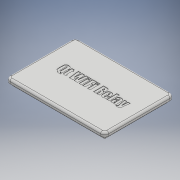
# Autodesk Inventor part: housing-lid
Saved by Autodesk Inventor 2018 (Build 220112000, 112)
## iProperties
Created: 2018-03-19
Part Number: housing-lid
Material: Generic
Document SubType Name: Modeling
Designer: matth
Density: 1 g/cm^3
Appearance: Default
Author: matth
Autodesk Inventor part; units mm, degrees
note: some values were not read from the file. Chosen so that the rebuilt part matches the saved one: direction of "Emboss1".
ref_plane "YZ Plane" through (0, 0, 0) normal (1, 0, 0) x (0, 1, 0)
ref_plane "XZ Plane" through (0, 0, 0) normal (0, 1, 0) x (-1, 0, 0)
ref_plane "XY Plane" through (0, 0, 0) normal (0, 0, 1) x (1, 0, 0)
sketch "Sketch1" plane through (0, 0, 0) normal (0, 0, 1) x (1, 0, 0)
  line L0 (0, 0) -> (46, 0)
  line L1 (46, 0) -> (46, 31.5)
  line L2 (46, 31.5) -> (0, 31.5)
  line L3 (0, 31.5) -> (0, 0)
  dimension "d0" = 46
  dimension "d1" = 31.5
  constraints: 8 end point, 2 parallel, 1 horizontal, 1 perpendicular
  measures "d0" distance of L1.end L2.end
  measures "d1" distance of L0.end L1.end
extrude "Extrusion1" add sketch "Sketch1" along normal blind 2
sketch "Sketch2" plane through (0, 0, 2) normal (0, 0, 1) x (1, 0, 0)
  line L0 (46, 0) -> (46, 31.5) projected
  line L1 (0, 0) -> (46, 0)
  line L2 (46, 0) -> (46, 31.5)
  line L3 (46, 31.5) -> (0, 31.5)
  line L4 (0, 31.5) -> (0, 0)
  line L5 (-1.4, 32.9) -> (47.4, 32.9)
  line L6 (47.4, 32.9) -> (47.4, -1.4)
  line L7 (47.4, -1.4) -> (-1.4, -1.4)
  line L8 (-1.4, -1.4) -> (-1.4, 32.9)
  dimension "d4" = 1.4
  constraints: 16 end point, 4 parallel, 2 perpendicular, 1 horizontal, 3 other
  measures "d4" distance between parallel lines of L3 L5
extrude "Extrusion2" add sketch "Sketch2" along normal blind 2 contours L1 L4 L3 L0 | L5 L6 L7 L8
sketch "Sketch3" plane through (0, 0, 0) normal (0, 0, -1) x (-1, 0, 0)
  line L0 (-46, 0) -> (-46, 31.5) projected
  line L1 (0, 0) -> (-46, 0)
  line L2 (-46, 0) -> (-46, 31.5)
  line L3 (-46, 31.5) -> (0, 31.5)
  line L4 (0, 31.5) -> (0, 0)
  line L5 (-43, 3) -> (-3, 3)
  line L6 (-3, 3) -> (-3, 28.5)
  line L7 (-3, 28.5) -> (-43, 28.5)
  line L8 (-43, 28.5) -> (-43, 3)
  dimension "d7" = 3
  constraints: 16 end point, 4 parallel, 2 perpendicular, 1 horizontal, 3 other
  measures "d7" distance between parallel lines of L1 L5
extrude "Extrusion3" cut sketch "Sketch3" against normal blind 2 contours L8 L7 L6 L5
chamfer "Chamfer1" distance 0.5 angle 45 4 edges at (23, 0, 0) (46, 15.75, 0) (23, 31.5, 0) (0, 15.75, 0)
chamfer "Chamfer2" distance 0.5 angle 45 4 edges at (0, 0, 1.25) (0, 31.5, 1.25) (46, 31.5, 1.25) (46, 0, 1.25)
fillet "Fillet1" radius 2 4 edges at (47.4, -1.4, 3) (47.4, 32.9, 3) (-1.4, 32.9, 3) (-1.4, -1.4, 3)
fillet "Fillet2" radius 1 8 edges at (46.8142, 32.3142, 4) (23, 32.9, 4) (-0.8142, 32.3142, 4) (-1.4, 15.75, 4) (-0.8142, -0.8142, 4) (23, -1.4, 4) (46.8142, -0.8142, 4) (47.4, 15.75, 4)
sketch "Sketch4" plane through (0, 0, 4) normal (0, 0, 1) x (1, 0, 0)
  line L0 (4.7033, 18.9978) -> (43.575, 18.9978) construction
  line L1 (43.575, 18.9978) -> (43.575, 6.6861) construction
  line L2 (43.575, 6.6861) -> (4.7033, 6.6861) construction
  line L3 (4.7033, 6.6861) -> (4.7033, 18.9978) construction
  line L4 (10.7801, 13.8923) -> (10.7801, 13.2857)
  line L5 (10.7801, 13.2857) -> (9.7967, 13.2857)
  spline S0 degree 2 poles (9.7967, 13.2857) (9.4425, 13.2857) (9.1524, 13.3949) (9.0506, 13.6135) (9.0506, 13.8923) knots 0 0 0 1 2 3 3 3
  spline S1 degree 2 poles (9.0506, 13.8923) (8.6098, 13.9036) (7.973, 14.3444) (7.7696, 15.0189) (7.7696, 15.6933) knots 0 0 0 1 2 3 3 3
  line L6 (7.7696, 15.6933) -> (7.7696, 17.242)
  spline S2 degree 2 poles (7.7696, 17.242) (7.7696, 17.7506) (7.8901, 18.2857) (8.2669, 18.7566) (8.8585, 18.9978) (9.2202, 18.9978) knots 0 0 0 1 2 3 4 4 4
  spline S3 degree 2 poles (9.2202, 18.9978) (9.6573, 18.9978) (10.3393, 18.7001) (10.6746, 18.2442) (10.7763, 17.7544) (10.7763, 17.2683) knots 0 0 0 1 2 3 4 4 4
  line L7 (10.7763, 17.2683) -> (10.7763, 15.6444)
  spline S4 degree 2 poles (10.7763, 15.6444) (10.7763, 14.9774) (10.6482, 14.5027) (10.279, 14.2201) (9.9738, 14.1485) knots 0 0 0 1 2 3 3 3
  spline S5 degree 2 poles (9.9738, 14.1485) (9.9813, 13.979) (10.1019, 13.8923) (10.328, 13.8923) knots 0 0 0 1 2 2 2
  line L8 (10.328, 13.8923) -> (10.7801, 13.8923)
  spline S6 degree 2 poles (9.4764, 17.6074) (9.4764, 17.9541) (9.4011, 18.15) (9.2805, 18.15) knots 0 0 0 1 2 2 2
  spline S7 degree 2 poles (9.2805, 18.15) (9.1787, 18.15) (9.0695, 17.9918) (9.0695, 17.6074) knots 0 0 0 1 2 2 2
  line L9 (9.0695, 17.6074) -> (9.0695, 15.2751)
  spline S8 degree 2 poles (9.0695, 15.2751) (9.0695, 14.838) (9.1411, 14.6346) (9.2692, 14.6346) knots 0 0 0 1 2 2 2
  spline S9 degree 2 poles (9.2692, 14.6346) (9.4011, 14.6346) (9.4764, 14.8682) (9.4764, 15.309) knots 0 0 0 1 2 2 2
  line L10 (9.4764, 15.309) -> (9.4764, 17.6074)
  line L11 (12.5397, 18.5381) -> (12.5397, 17.8938)
  line L12 (12.5397, 17.8938) -> (12.8788, 17.8938)
  line L13 (12.8788, 17.8938) -> (12.8788, 17.2457)
  line L14 (12.8788, 17.2457) -> (12.5397, 17.2457)
  line L15 (12.5397, 17.2457) -> (12.5397, 15.049)
  spline S10 degree 2 poles (12.5397, 15.049) (12.5397, 14.6459) (12.6226, 14.5517) (12.9316, 14.5517) knots 0 0 0 1 2 2 2
  line L16 (12.9316, 14.5517) -> (12.9316, 13.8923)
  line L17 (12.9316, 13.8923) -> (12.4267, 13.8923)
  spline S11 degree 2 poles (12.4267, 13.8923) (12.0009, 13.8923) (11.6354, 13.9639) (11.3566, 14.2201) (11.2888, 14.5517) (11.2888, 15.1621) knots 0 0 0 1 2 3 4 4 4
  line L18 (11.2888, 15.1621) -> (11.2888, 17.2457)
  line L19 (11.2888, 17.2457) -> (11.0212, 17.2457)
  line L20 (11.0212, 17.2457) -> (11.0212, 17.8938)
  line L21 (11.0212, 17.8938) -> (11.2888, 17.8938)
  line L22 (11.2888, 17.8938) -> (11.2888, 18.5381)
  line L23 (11.2888, 18.5381) -> (12.5397, 18.5381)
  line L24 (19.1976, 18.8923) -> (18.6173, 13.8923)
  line L25 (18.6173, 13.8923) -> (16.9971, 13.8923)
  spline S12 degree 2 poles (16.9971, 13.8923) (16.7748, 15.0453) (16.6053, 16.5147) knots 0 0 0 1 1 1
  spline S13 degree 2 poles (16.6053, 16.5147) (16.5224, 15.8855) (16.2398, 13.8923) knots 0 0 0 1 1 1
  line L26 (16.2398, 13.8923) -> (14.6271, 13.8923)
  line L27 (14.6271, 13.8923) -> (14.0469, 18.8923)
  line L28 (14.0469, 18.8923) -> (15.3091, 18.8923)
  line L29 (15.3091, 18.8923) -> (15.4448, 17.1478)
  line L30 (15.4448, 17.1478) -> (15.5804, 15.4597)
  spline S14 degree 2 poles (15.5804, 15.4597) (15.652, 16.771) (15.9384, 18.8923) knots 0 0 0 1 1 1
  line L31 (15.9384, 18.8923) -> (17.2873, 18.8923)
  spline S15 degree 2 poles (17.2873, 18.8923) (17.3136, 18.6738) (17.4267, 17.242) knots 0 0 0 1 1 1
  line L32 (17.4267, 17.242) -> (17.5736, 15.3392)
  spline S16 degree 2 poles (17.5736, 15.3392) (17.6867, 17.1553) (17.9353, 18.8923) knots 0 0 0 1 1 1
  line L33 (17.9353, 18.8923) -> (19.1976, 18.8923)
  line L34 (20.7047, 17.9918) -> (20.7047, 13.8923)
  line L35 (20.7047, 13.8923) -> (19.4199, 13.8923)
  line L36 (19.4199, 13.8923) -> (19.4199, 17.9918)
  line L37 (19.4199, 17.9918) -> (20.7047, 17.9918)
  line L38 (20.7047, 18.8923) -> (20.7047, 18.2404)
  line L39 (20.7047, 18.2404) -> (19.4199, 18.2404)
  line L40 (19.4199, 18.2404) -> (19.4199, 18.8923)
  line L41 (19.4199, 18.8923) -> (20.7047, 18.8923)
  line L42 (21.1908, 18.8923) -> (23.3913, 18.8923)
  line L43 (23.3913, 18.8923) -> (23.3913, 17.89)
  line L44 (23.3913, 17.89) -> (22.4907, 17.89)
  line L45 (22.4907, 17.89) -> (22.4907, 16.9443)
  line L46 (22.4907, 16.9443) -> (23.2933, 16.9443)
  line L47 (23.2933, 16.9443) -> (23.2933, 15.991)
  line L48 (23.2933, 15.991) -> (22.4907, 15.991)
  line L49 (22.4907, 15.991) -> (22.4907, 13.8923)
  line L50 (22.4907, 13.8923) -> (21.1908, 13.8923)
  line L51 (21.1908, 13.8923) -> (21.1908, 18.8923)
  line L52 (24.9549, 17.9918) -> (24.9549, 13.8923)
  line L53 (24.9549, 13.8923) -> (23.6701, 13.8923)
  line L54 (23.6701, 13.8923) -> (23.6701, 17.9918)
  line L55 (23.6701, 17.9918) -> (24.9549, 17.9918)
  line L56 (24.9549, 18.8923) -> (24.9549, 18.2404)
  line L57 (24.9549, 18.2404) -> (23.6701, 18.2404)
  line L58 (23.6701, 18.2404) -> (23.6701, 18.8923)
  line L59 (23.6701, 18.8923) -> (24.9549, 18.8923)
  line L60 (26.5563, 18.8923) -> (27.4757, 18.8923)
  spline S17 degree 2 poles (27.4757, 18.8923) (28.395, 18.8923) (29.0469, 18.7491) (29.4576, 18.1651) (29.4576, 17.5283) knots 0 0 0 1 2 3 3 3
  spline S18 degree 2 poles (29.4576, 17.5283) (29.4576, 16.9443) (29.1674, 16.5411) (28.7417, 16.4997) knots 0 0 0 1 2 2 2
  spline S19 degree 2 poles (28.7417, 16.4997) (29.126, 16.4055) (29.3935, 16.0852) (29.4576, 15.8177) (29.4576, 15.2111) knots 0 0 0 1 2 3 3 3
  line L61 (29.4576, 15.2111) -> (29.4576, 13.8923)
  line L62 (29.4576, 13.8923) -> (28.2481, 13.8923)
  line L63 (28.2481, 13.8923) -> (28.2481, 15.5539)
  spline S20 degree 2 poles (28.2481, 15.5539) (28.2481, 15.9533) (28.1237, 16.1455) (27.8562, 16.1455) knots 0 0 0 1 2 2 2
  line L64 (27.8562, 16.1455) -> (27.8562, 13.8923)
  line L65 (27.8562, 13.8923) -> (26.5563, 13.8923)
  line L66 (26.5563, 13.8923) -> (26.5563, 18.8923)
  line L67 (27.8562, 18.037) -> (27.8562, 16.9254)
  spline S21 degree 2 poles (27.8562, 16.9254) (28.0748, 16.9254) (28.2481, 17.046) (28.2481, 17.3776) knots 0 0 0 1 2 2 2
  line L68 (28.2481, 17.3776) -> (28.2481, 17.6527)
  spline S22 degree 2 poles (28.2481, 17.6527) (28.2481, 17.89) (28.0785, 18.037) (27.8562, 18.037) knots 0 0 0 1 2 2 2
  line L69 (32.7507, 15.8704) -> (31.1343, 15.8704)
  line L70 (31.1343, 15.8704) -> (31.1343, 14.985)
  spline S23 degree 2 poles (31.1343, 14.985) (31.1343, 14.7062) (31.2134, 14.5441) (31.3302, 14.5441) knots 0 0 0 1 2 2 2
  spline S24 degree 2 poles (31.3302, 14.5441) (31.4734, 14.5441) (31.5676, 14.7589) (31.5676, 15.0641) knots 0 0 0 1 2 2 2
  line L71 (31.5676, 15.0641) -> (31.5676, 15.6029)
  line L72 (31.5676, 15.6029) -> (32.7507, 15.6029)
  line L73 (32.7507, 15.6029) -> (32.7507, 15.3015)
  spline S25 degree 2 poles (32.7507, 15.3015) (32.7507, 14.9209) (32.6565, 14.514) (32.3023, 14.0505) (31.7635, 13.8169) (31.3528, 13.8169) knots 0 0 0 1 2 3 4 4 4
  spline S26 degree 2 poles (31.3528, 13.8169) (30.9572, 13.8169) (30.3543, 14.0468) (30.0152, 14.4462) (29.8871, 14.9247) (29.8871, 15.3806) knots 0 0 0 1 2 3 4 4 4
  line L74 (29.8871, 15.3806) -> (29.8871, 16.5788)
  spline S27 degree 2 poles (29.8871, 16.5788) (29.8871, 17.1138) (30.1772, 17.7355) (30.8404, 18.0671) (31.2662, 18.0671) knots 0 0 0 1 2 3 3 3
  spline S28 degree 2 poles (31.2662, 18.0671) (31.7937, 18.0671) (32.4757, 17.6677) (32.7507, 17.0121) (32.7507, 16.413) knots 0 0 0 1 2 3 3 3
  line L75 (32.7507, 16.413) -> (32.7507, 15.8704)
  line L76 (31.4998, 16.5374) -> (31.4998, 16.835)
  spline S29 degree 2 poles (31.4998, 16.835) (31.4998, 17.1553) (31.4319, 17.3399) (31.3264, 17.3399) knots 0 0 0 1 2 2 2
  spline S30 degree 2 poles (31.3264, 17.3399) (31.1946, 17.3399) (31.1343, 17.1817) (31.1343, 16.835) knots 0 0 0 1 2 2 2
  line L77 (31.1343, 16.835) -> (31.1343, 16.5374)
  line L78 (31.1343, 16.5374) -> (31.4998, 16.5374)
  line L79 (34.4425, 18.8923) -> (34.4425, 13.8923)
  line L80 (34.4425, 13.8923) -> (33.1576, 13.8923)
  line L81 (33.1576, 13.8923) -> (33.1576, 18.8923)
  line L82 (33.1576, 18.8923) -> (34.4425, 18.8923)
  line L83 (36.0062, 16.4055) -> (34.8344, 16.4055)
  line L84 (34.8344, 16.4055) -> (34.8344, 16.6805)
  spline S31 degree 2 poles (34.8344, 16.6805) (34.8344, 17.1553) (35.0529, 17.6715) (35.716, 18.0671) (36.2436, 18.0671) knots 0 0 0 1 2 3 3 3
  spline S32 degree 2 poles (36.2436, 18.0671) (36.8766, 18.0671) (37.5209, 17.6187) (37.649, 16.9669) (37.649, 15.9496) knots 0 0 0 1 2 3 3 3
  line L85 (37.649, 15.9496) -> (37.649, 13.8923)
  line L86 (37.649, 13.8923) -> (36.4357, 13.8923)
  line L87 (36.4357, 13.8923) -> (36.4357, 14.2578)
  spline S33 degree 2 poles (36.4357, 14.2578) (36.3227, 14.0392) (35.961, 13.8169) (35.7085, 13.8169) knots 0 0 0 1 2 2 2
  spline S34 degree 2 poles (35.7085, 13.8169) (35.3807, 13.8169) (34.8344, 14.1862) (34.8344, 14.8079) knots 0 0 0 1 2 2 2
  line L88 (34.8344, 14.8079) -> (34.8344, 15.1432)
  spline S35 degree 2 poles (34.8344, 15.1432) (34.8344, 15.6029) (35.1245, 15.9383) (35.701, 16.1606) knots 0 0 0 1 2 2 2
  spline S36 degree 2 poles (35.701, 16.1606) (36.3151, 16.4017) (36.4018, 16.5675) (36.4018, 16.8237) knots 0 0 0 1 2 2 2
  spline S37 degree 2 poles (36.4018, 16.8237) (36.4018, 17.144) (36.3076, 17.3399) (36.1946, 17.3399) knots 0 0 0 1 2 2 2
  spline S38 degree 2 poles (36.1946, 17.3399) (36.0665, 17.3399) (36.0062, 17.1779) (36.0062, 16.835) knots 0 0 0 1 2 2 2
  line L89 (36.0062, 16.835) -> (36.0062, 16.4055)
  spline S39 degree 2 poles (36.4018, 15.8441) (36.1004, 15.6255) (36.0062, 15.3279) (36.0062, 15.049) knots 0 0 0 1 2 2 2
  spline S40 degree 2 poles (36.0062, 15.049) (36.0062, 14.7288) (36.0891, 14.5441) (36.2134, 14.5441) knots 0 0 0 1 2 2 2
  spline S41 degree 2 poles (36.2134, 14.5441) (36.3302, 14.5441) (36.4018, 14.6911) (36.4018, 15.0001) knots 0 0 0 1 2 2 2
  line L90 (36.4018, 15.0001) -> (36.4018, 15.8441)
  line L91 (40.6934, 17.9918) -> (40.3355, 15.0264)
  spline S42 degree 2 poles (40.3355, 15.0264) (40.2488, 14.3218) (40.1358, 13.8094) (39.872, 13.4778) (39.3973, 13.3196) (38.8773, 13.3196) knots 0 0 0 1 2 3 4 4 4
  line L92 (38.8773, 13.3196) -> (38.12, 13.3196)
  line L93 (38.12, 13.3196) -> (38.12, 13.9752)
  spline S43 degree 2 poles (38.12, 13.9752) (38.4139, 13.9752) (38.5797, 14.0355) (38.5797, 14.1372) knots 0 0 0 1 2 2 2
  spline S44 degree 2 poles (38.5797, 14.1372) (38.5797, 14.1862) (38.5043, 14.5667) knots 0 0 0 1 1 1
  line L94 (38.5043, 14.5667) -> (37.8185, 17.9918)
  line L95 (37.8185, 17.9918) -> (38.9527, 17.9918)
  line L96 (38.9527, 17.9918) -> (39.3634, 15.2224)
  line L97 (39.3634, 15.2224) -> (39.5593, 17.9918)
  line L98 (39.5593, 17.9918) -> (40.6934, 17.9918)
  point P0 (0, 0)
  constraints: 2 other
emboss "Emboss1" sketch "Sketch4" operation cut depth 0.2 direction (0, 0, -1)
body "Solid1"
